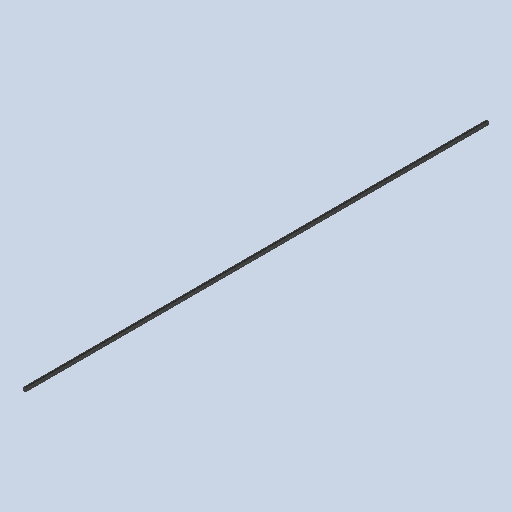
# Autodesk Inventor part: BSH 064 tube 4
Saved by Autodesk Inventor 2025 (Build 290162010, 162A)
## iProperties
Created: 2024-07-30
Part Number: BSH 064 tube 4
Material: Steel
Document SubType Name: Modeling
Designer: pokla
Density: 7.85 g/cm^3
Appearance: Plate
Author: pokla
Autodesk Inventor part; units mm, degrees
ref_plane "YZ Plane" through (0, 0, 0) normal (1, 0, 0) x (0, 1, 0)
ref_plane "XZ Plane" through (0, 0, 0) normal (0, 1, 0) x (-1, 0, 0)
ref_plane "XY Plane" through (0, 0, 0) normal (0, 0, 1) x (1, 0, 0)
sketch "Sketch1" plane through (0, 0, 0) normal (0, 1, 0) x (-1, 0, 0)
  line L0 (-25, -19) -> (-25, 19)
  line L1 (-19, 25) -> (19, 25)
  line L2 (25, 19) -> (25, -19)
  line L3 (19, -25) -> (-19, -25)
  arc A0 (-25, -19) -> (-19, -25) centre (-19, -19) ccw
  arc A1 (25, 19) -> (19, 25) centre (19, 19) ccw
  arc A2 (-19, 25) -> (-25, 19) centre (-19, 19) ccw
  arc A3 (19, -25) -> (25, -19) centre (19, -19) ccw
  arc A4 (-19, 23) -> (-23, 19) centre (-19, 19) ccw
  line L4 (-19, 23) -> (19, 23)
  arc A5 (23, 19) -> (19, 23) centre (19, 19) ccw
  line L5 (23, 19) -> (23, -19)
  arc A6 (19, -23) -> (23, -19) centre (19, -19) ccw
  line L6 (19, -23) -> (-19, -23)
  arc A7 (-23, -19) -> (-19, -23) centre (-19, -19) ccw
  line L7 (-23, -19) -> (-23, 19)
  line L8 (0, 25) -> (0, -25) construction
  point P0 (0, 0)
  point P1 (0, 0)
  dimension "d0" = 6
  dimension "d1" = 50
  dimension "d2" = 50
  dimension "d3" = 2
  constraints: 18 end point, 16 point on circle, 8 centre point, 8 tangent, 4 parallel, 3 equal radius, 3 midpoint, 2 perpendicular, 1 coincident, 1 vertical, 7 other
  measures "d0" radius of A0
  measures "d1" distance between parallel lines of L0 L2
  measures "d2" distance between parallel lines of L1 L3
  measures "d3" distance between parallel lines of L2 L5
extrude "Extrusion1" add sketch "Sketch1" along normal mid plane 8080
equation "\"d6\" = 6"
equation "\"d9\" = 3"
body "Solid1"
